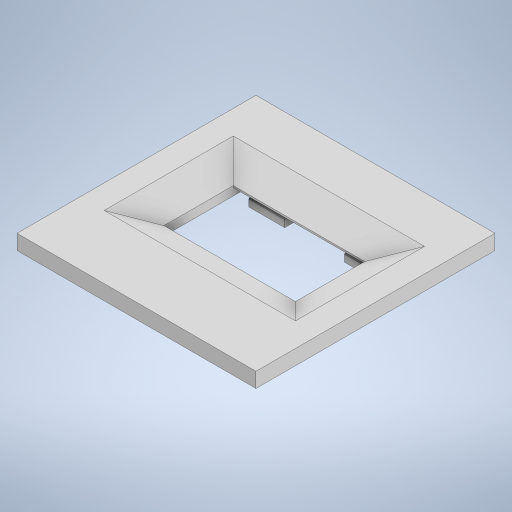
# Autodesk Inventor part: DisplayInsert
Saved by Autodesk Inventor 2024 (Build 280153000, 153)
## iProperties
Created: 2025-09-20
Part Number: DisplayInsert
Material: Generic
Document SubType Name: Modeling
Designer: Martin
Density: 1 g/cm^3
Appearance: Default
Author: Martin
Autodesk Inventor part; units mm, degrees
ref_plane "YZ Plane" through (0, 0, 0) normal (1, 0, 0) x (0, 1, 0)
ref_plane "XZ Plane" through (0, 0, 0) normal (0, 1, 0) x (-1, 0, 0)
ref_plane "XY Plane" through (0, 0, 0) normal (0, 0, 1) x (1, 0, 0)
sketch "Sketch1" plane through (0, 0, 0) normal (0, 1, 0) x (-1, 0, 0)
  line L0 (-25.4, 25.4) -> (25.4, 25.4)
  line L1 (25.4, 25.4) -> (25.4, -25.4)
  line L2 (25.4, -25.4) -> (-25.4, -25.4)
  line L3 (-25.4, -25.4) -> (-25.4, 25.4)
  line L4 (-25.4, 25.4) -> (25.4, -25.4) construction
  line L5 (25.4, 25.4) -> (-25.4, -25.4) construction
  point P0 (0, 0)
  dimension "d0" = 50.8
  dimension "d1" = 50.8
  constraints: 12 end point, 2 midpoint, 2 parallel, 1 horizontal, 1 perpendicular
  measures "d0" distance of L1.end L2.end
  measures "d1" distance of L0.end L1.end
extrude "Extrusion1" add sketch "Sketch1" along normal blind 3.175
sketch "Sketch2" plane through (0, 0, 0) normal (0, -1, 0) x (1, 0, 0)
  line L0 (-11.811, 11.811) -> (11.811, 11.811) construction
  line L1 (11.811, 11.811) -> (11.811, -11.811) construction
  line L2 (11.811, -11.811) -> (-11.811, -11.811) construction
  line L3 (-11.811, -11.811) -> (-11.811, 11.811) construction
  circle A0 centre (-11.811, 11.811) radius 0.9525
  line L4 (13.97, 13.97) -> (-13.97, 13.97) construction
  line L5 (-13.97, 13.97) -> (-13.97, -13.97) construction
  line L6 (-13.97, -13.97) -> (13.97, -13.97) construction
  line L7 (13.97, -13.97) -> (13.97, 13.97) construction
  line L8 (13.97, 13.97) -> (6.35, 13.97)
  line L9 (6.35, 13.97) -> (6.35, 10.16)
  line L10 (6.35, 10.16) -> (13.97, 10.16)
  line L11 (13.97, 10.16) -> (13.97, 13.97)
  line L12 (-13.97, 13.97) -> (-6.35, 13.97)
  line L13 (-6.35, 13.97) -> (-6.35, 10.16)
  line L14 (-6.35, 10.16) -> (-13.97, 10.16)
  line L15 (-13.97, 10.16) -> (-13.97, 13.97)
  circle A1 centre (11.811, 11.811) radius 0.9525
  line L16 (13.97, 13.97) -> (18.034, 13.97)
  line L17 (18.034, 13.97) -> (18.034, -17.526)
  line L18 (18.034, -17.526) -> (13.97, -17.526)
  line L19 (13.97, -17.526) -> (13.97, 13.97)
  line L20 (-13.97, 13.97) -> (-18.034, 13.97)
  line L21 (-18.034, 13.97) -> (-18.034, -17.526)
  line L22 (-18.034, -17.526) -> (-13.97, -17.526)
  line L23 (-13.97, -17.526) -> (-13.97, 13.97)
  point P0 (0, 0)
  point P1 (11.811, 0)
  point P2 (0, 11.811)
  point P3 (0, -13.97)
  point P4 (-13.97, 0)
  point P5 (-13.97, 10.16)
  point P6 (13.97, 10.16)
  dimension "d4" = 23.622
  dimension "d5" = 23.622
  dimension "d27" = 27.94
  dimension "d28" = 27.94
  dimension "d29" = 7.62
  dimension "d30" = 3.81
  dimension "d31" = 1.905
  dimension "d32" = 4.064
  dimension "d33" = 4.064
  dimension "d46" = 31.496
  constraints: 48 end point, 12 parallel, 6 horizontal, 6 perpendicular, 4 midpoint, 3 equal length, 2 centre point, 2 coincident, 2 horizontal alignment, 2 vertical alignment, 1 equal radius
  measures "d4" distance of L1.end L2.end
  measures "d5" distance of L0.end L1.end
  measures "d27" distance of L5.end L6.end
  measures "d28" distance of L4.end L5.end
  measures "d29" distance of L10.end L9.end
  measures "d30" distance of L8.end L9.end
  measures "d31" diameter of A1
  measures "d32" distance of L17.end L18.end
  measures "d33" distance of L22.end L21.end
  measures "d46" distance of L20.end L21.end
extrude "Extrusion2" add sketch "Sketch2" along normal blind 1.524
sketch "Sketch3" plane through (0, 0, 0) normal (0, -1, 0) x (1, 0, 0)
  line L0 (13.97, 13.97) -> (-13.97, 13.97) construction
  line L1 (-13.97, 13.97) -> (-13.97, -13.97) construction
  line L2 (-13.97, -13.97) -> (13.97, -13.97) construction
  line L3 (13.97, -13.97) -> (13.97, 13.97) construction
  line L4 (13.97, 13.97) -> (-13.97, -13.97) construction
  line L5 (-13.97, 13.97) -> (13.97, -13.97) construction
  line L6 (13.97, 5.588) -> (-13.97, 5.588)
  line L7 (-13.97, 5.588) -> (-13.97, -9.144)
  line L8 (-13.97, -9.144) -> (13.97, -9.144)
  line L9 (13.97, -9.144) -> (13.97, 5.588)
  point P0 (0, 0)
  dimension "d18" = 27.94
  dimension "d19" = 27.94
  dimension "d20" = 4.826
  dimension "d21" = 14.732
  constraints: 20 end point, 4 parallel, 2 horizontal, 2 midpoint, 2 perpendicular, 2 point on line
  measures "d18" distance of L2.end L1.end
  measures "d19" distance of L1.end L0.end
  measures "d20" distance between parallel lines of L8 L2
  measures "d21" distance between parallel lines of L6 L8
sketch "Sketch4" plane through (0, 3.175, 0) normal (0, 1, 0) x (1, 0, 0)
  line L0 (-13.97, 9.144) -> (13.97, 9.144) projected
  line L1 (13.97, -5.588) -> (-13.97, -5.588) projected
  line L2 (-13.97, -5.588) -> (-13.97, 9.144) projected
  line L3 (13.97, 9.144) -> (13.97, -5.588) projected
  line L4 (-20.32, -11.938) -> (20.32, -11.938)
  line L5 (20.32, -11.938) -> (20.32, 15.494)
  line L6 (20.32, 15.494) -> (-20.32, 15.494)
  line L7 (-20.32, 15.494) -> (-20.32, -11.938)
  point P0 (0, 0)
  dimension "d22" = 6.35
  constraints: 8 end point, 3 other
  measures "d22" distance between parallel lines of L1 L4
sketch "Sketch5" plane through (0, 0, 0) normal (1, 0, 0) x (0, 1, 0)
  line L0 (0, 25.4) -> (0, -25.4) projected
  line L1 (0, -12.446) -> (-1.524, -12.446)
  line L2 (-1.524, 10.16) -> (-1.524, -17.526) projected
  line L3 (-1.524, -12.446) -> (-1.524, -13.97)
  line L4 (-1.524, -13.97) -> (-2.794, -13.97)
  line L5 (-2.794, -13.97) -> (-3.6739, -12.446)
  line L6 (-3.6739, -12.446) -> (-5.1979, -12.446)
  line L7 (-5.1979, -12.446) -> (-5.1979, -17.526)
  line L8 (-5.1979, -17.526) -> (0, -17.526)
  line L9 (0, -17.526) -> (0, -12.446)
  line L10 (3.175, -16.002) -> (3.175, 11.43) projected
  line L11 (0, 13.97) -> (-1.524, 13.97) projected
  point P0 (0, 0)
  point P1 (0, -17.526)
  dimension "d34" = 1.524
  dimension "d35" = 1.524
  dimension "d36" = 1.27
  dimension "d37" = 120
  dimension "d38" = 1.524
  dimension "d39" = 5.08
  dimension "d40" = 27.94
  constraints: 16 end point, 4 perpendicular, 4 point on line, 1 collinear
  measures "d34" distance of L1.start L1.end
  measures "d35" distance of L1.end L3.end
  measures "d36" distance of L3.end L4.end
  measures "d37" angle of L4 L5
  measures "d38" distance of L5.end L6.end
  measures "d39" distance of L6.end L7.end
  measures "d40" distance between parallel lines of L4 L11
extrude "Extrusion3" add sketch "Sketch5" along normal mid plane 27.94
sketch "Sketch6" plane through (0, 0, 0) normal (0, -1, 0) x (1, 0, 0)
  line L0 (-13.97, -17.526) -> (13.97, -17.526) projected
  line L1 (13.97, -12.446) -> (13.97, -17.526) projected
  line L2 (-13.97, -12.446) -> (13.97, -12.446) projected
  line L3 (-13.97, -17.526) -> (-13.97, -12.446) projected
  line L4 (-6.35, -12.446) -> (6.35, -12.446)
  line L5 (6.35, -12.446) -> (6.35, -17.526)
  line L6 (6.35, -17.526) -> (-6.35, -17.526)
  line L7 (-6.35, -17.526) -> (-6.35, -12.446)
  point P0 (0, 0)
  point P1 (0, -12.446)
  point P2 (0, -12.446)
  dimension "d43" = 12.7
  constraints: 8 end point, 2 midpoint, 2 parallel, 2 point on line, 1 coincident, 1 horizontal, 1 perpendicular
  measures "d43" distance of L5.end L6.end
extrude "Extrusion4" cut sketch "Sketch6" along normal up to surface (5.1979 mm away) contours L7 L2 L5 L0
sketch "Sketch7" plane through (0, 0, 0) normal (0, -1, 0) x (1, 0, 0)
  circle A0 centre (11.811, 11.811) radius 0.9525 projected
  circle A1 centre (-11.811, 11.811) radius 0.9525 projected
  point P0 (0, 0)
extrude "Extrusion5" cut sketch "Sketch7" against normal blind 2.54
extrude "Extrusion7" cut sketch "Sketch3" against normal blind 0.381
loft "Loft2" cut profiles "Sketch4" section 1 edges at (-13.97, 0.381, -1.778) (0, 0.381, -9.144) (13.97, 0.381, -1.778) (0, 0.381, 5.588) contours L0 L3 L1 L2 | L7 L6 L5 L4
body "Solid1"
